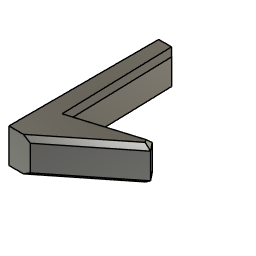
Hooks v1 (Autodesk Fusion 360 design; units mm, degrees)
Autodesk Fusion 360 part; units mm, degrees
sketch "Sketch1" plane through (0, 0, 0) normal (0, 0, 1) x (1, 0, 0)
  line L0 (0, 0) -> (0, 70)
  line L1 (0, 0) -> (10, 0)
  line L2 (10, 0) -> (41.3229, 24.8773)
  line L3 (0, 70) -> (8, 70)
  line L4 (8, 70) -> (9.428, 20.0204)
  line L5 (41.3229, 24.8773) -> (38.2132, 28.7926)
  line L6 (9.428, 20.0204) -> (38.2132, 28.7926)
  dimension "d2" = 70
  dimension "d3" = 10
  dimension "d4" = 40
  dimension "d5" = 8
  dimension "d6" = 50
  dimension "d7" = 5
  constraint coincident L0.start L1.start
  constraint vertical L0
  constraint perpendicular L0 L1
  constraint perpendicular L0 L3
  constraint perpendicular L2 L5
  measures "d2" distance of L0.start L0.end
  measures "d3" distance of L0.start L1.end
  measures "d4" distance of L1.end L2.end
  measures "d5" distance of L0.end L3.end
  measures "d6" distance of L3.end L4.end
  measures "d7" distance of L2.end L5.end
extrude "Extrude1" add sketch "Sketch1" along normal blind 16
chamfer "Chamfer1" distance 2 angle 45 13 edges at (8.714, 45.0102, 16) (23.8206, 24.4065, 16) (25.6614, 12.4386, 16) (39.768, 26.8349, 16) (5, 0, 16) (4, 70, 16) (8, 70, 8) (25.6614, 12.4386, 0) (5, 0, 0) (39.768, 26.8349, 0) (23.8206, 24.4065, 0) (8.714, 45.0102, 0) (4, 70, 0)
delete_face "DeleteFace1" 1 faces at (4.0188, 68.6667, 15.3333)
delete_face "DeleteFace2" 1 faces at (5.3516, 69.3333, 15.3333)
delete_face "DeleteFace3" 2 faces at (6.7045, 68.6669, 1.3333) (4.0188, 68.6667, 0.6667)
delete_face "DeleteFace4" 2 faces at (6.4341, 0.6667, 14.6667) (6.4341, 0.6667, 1.3333)
